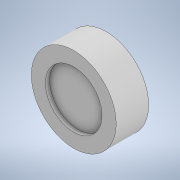
# Autodesk Inventor part: roue
Saved by Autodesk Inventor 2020 (Build 240168000, 168)
## iProperties
Created: 2024-02-01
Part Number: roue
Material: Générique
Document SubType Name: Modeling
Designer: Stark
Density: 1 g/cm^3
Appearance: Par défaut
Author: Stark
Autodesk Inventor part; units mm, degrees
ref_plane "YZ Plane" through (0, 0, 0) normal (1, 0, 0) x (0, 1, 0)
ref_plane "XZ Plane" through (0, 0, 0) normal (0, 1, 0) x (-1, 0, 0)
ref_plane "XY Plane" through (0, 0, 0) normal (0, 0, 1) x (1, 0, 0)
sketch "Esquisse2" plane through (0, 0, 0) normal (0, 0, 1) x (1, 0, 0)
  circle A0 centre (0, 0) radius 300
  dimension "d3" = 600
  constraints: 1 centre point, 1 coincident
  measures "d3" diameter of A0
extrude "Extrusion2" add sketch "Esquisse2" along normal blind 230
sketch "Esquisse3" plane through (0, 0, 230) normal (0, 0, 1) x (1, 0, 0)
  circle A0 centre (0, 0) radius 200
  dimension "d6" = 400
  constraints: 1 centre point, 1 coincident
  measures "d6" diameter of A0
extrude "Extrusion3" cut sketch "Esquisse3" against normal blind 30
sketch "Esquisse4" plane through (0, 0, 0) normal (0, 0, -1) x (-1, 0, 0)
  circle A0 centre (0, 0) radius 200
  dimension "d9" = 400
  constraints: 1 centre point, 1 coincident
  measures "d9" diameter of A0
extrude "Extrusion4" cut sketch "Esquisse4" against normal blind 30
